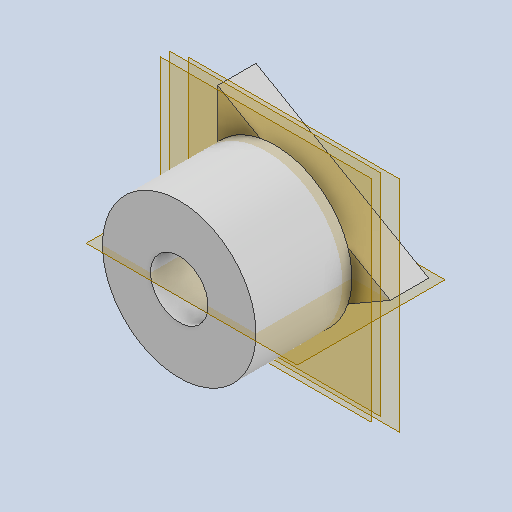
# Autodesk Inventor part: handle_base_potholder
Saved by Autodesk Inventor 2022 (Build 260153000, 153)
## iProperties
Created: 2021-07-05
Part Number: handle_base_potholder
Material: Generic
Document SubType Name: Modeling
Designer: teh18
Density: 1 g/cm^3
Appearance: Default
Author: teh18
Autodesk Inventor part; units mm, degrees
ref_plane "YZ Plane" through (0, 0, 0) normal (1, 0, 0) x (0, 1, 0)
ref_plane "Work Plane1" through (0, 0, 0) normal (0, 0, 1) x (1, 0, 0)
sketch "Sketch2" plane through (0, 0, 0) normal (0, 0, 1) x (1, 0, 0)
  line L0 (5.0552, -5.3443) -> (3.4937, -4.879) projected
  arc A0 (0.6492, -5.9656) -> (3.4937, -4.879) centre (0, 0) ccw projected
  line L1 (0.6492, -5.9656) -> (-0.2044, -7.3536) projected
  line L2 (-0.2044, -7.3536) -> (-0.9796, -5.9204) projected
  arc A1 (-3.7593, -4.6774) -> (-0.9796, -5.9204) centre (0, 0) ccw projected
  line L3 (-3.7593, -4.6774) -> (-5.3443, -5.0552) projected
  line L4 (-5.3443, -5.0552) -> (-4.879, -3.4937) projected
  arc A2 (-5.9656, -0.6492) -> (-4.879, -3.4937) centre (0, 0) ccw projected
  line L5 (-5.9656, -0.6492) -> (-7.3536, 0.2044) projected
  line L6 (-7.3536, 0.2044) -> (-5.9204, 0.9796) projected
  arc A3 (-4.6774, 3.7593) -> (-5.9204, 0.9796) centre (0, 0) ccw projected
  line L7 (-4.6774, 3.7593) -> (-5.0552, 5.3443) projected
  line L8 (-5.0552, 5.3443) -> (-3.4937, 4.879) projected
  arc A4 (-0.6492, 5.9656) -> (-3.4937, 4.879) centre (0, 0) ccw projected
  line L9 (-0.6492, 5.9656) -> (0.2044, 7.3536) projected
  line L10 (0.2044, 7.3536) -> (0.9796, 5.9204) projected
  arc A5 (3.7593, 4.6774) -> (0.9796, 5.9204) centre (0, 0) ccw projected
  line L11 (3.7593, 4.6774) -> (5.3443, 5.0552) projected
  line L12 (5.3443, 5.0552) -> (4.879, 3.4937) projected
  arc A6 (5.9656, 0.6492) -> (4.879, 3.4937) centre (0, 0) ccw projected
  line L13 (5.9656, 0.6492) -> (7.3536, -0.2044) projected
  line L14 (7.3536, -0.2044) -> (5.9204, -0.9796) projected
  arc A7 (4.6774, -3.7593) -> (5.9204, -0.9796) centre (0, 0) ccw projected
  line L15 (4.6774, -3.7593) -> (5.0552, -5.3443) projected
  circle A8 centre (0, 0) radius 3
  line L16 (-3, 0.5) -> (3, 0.5)
  line L17 (3, 0.5) -> (3, -0.5)
  line L18 (3, -0.5) -> (-3, -0.5)
  line L19 (-3, -0.5) -> (-3, 0.5)
  line L20 (-3, 0.5) -> (3, -0.5) construction
  line L21 (3, 0.5) -> (-3, -0.5) construction
  circle A9 centre (0, 0) radius 18 projected
  point P0 (0, 0)
  point P1 (-3, 0)
  point P2 (-2.958, 0.5)
  point P3 (2.958, 0.5)
  point P4 (3, 0)
  point P5 (2.958, -0.5)
  point P6 (-2.958, -0.5)
  dimension "d2" = 6
  dimension "d3" = 6
  dimension "d4" = 1
  constraints: 12 end point, 2 midpoint, 2 parallel, 1 centre point, 1 horizontal, 1 perpendicular
  measures "d2" diameter of A8
  measures "d3" distance of L17.end L18.end
  measures "d4" distance of L16.end L17.end
extrude "Extrusion2" add sketch "Sketch2" along normal blind 1 contours A8 L18 L16
ref_plane "Work Plane2" through (0, 0, 1) normal (0, 0, 1) x (0, -1, 0)
sketch "Sketch3" plane through (0, 0, 0) normal (0, 0, 1) x (0, -1, 0)
  circle A0 centre (0, 0) radius 8 projected
  arc A1 (0.5, -2.958) -> (0.5, 2.958) centre (0, 0) ccw projected
  line L0 (0.5, -2.958) -> (0.5, 2.958) projected
  line L1 (-0.5, 2.958) -> (-0.5, -2.958) projected
  arc A2 (-0.5, 2.958) -> (-0.5, -2.958) centre (0, 0) ccw projected
  circle A3 centre (0, 0) radius 3
  point P0 (0, 0)
  point P1 (0.5, -2.958)
  point P2 (-0.5, -2.958)
  point P3 (-0.5, 2.958)
  point P4 (3, 0)
  constraints: 1 centre point, 1 coincident
extrude "Extrusion3" add sketch "Sketch3" along normal blind 10
sketch "Sketch4" plane through (0, 0, 0) normal (0, 0, 1) x (1, 0, 0)
  circle A0 centre (0, 0) radius 6
  line L0 (-6, 10.3923) -> (12, 0)
  line L1 (12, 0) -> (-6, -10.3923)
  line L2 (-6, -10.3923) -> (-6, 10.3923)
  point P0 (-6, 0)
  point P1 (3, -5.1962)
  point P2 (3, 5.1962)
  dimension "d9" = 12
  constraints: 6 end point, 3 coincident, 1 midpoint, 10 other
extrude "Extrusion4" add sketch "Sketch4" against normal blind 4
body "Solid1"
